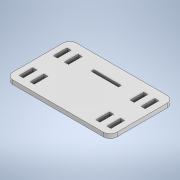
# Autodesk Inventor part: cambase
Saved by Autodesk Inventor 2020 (Build 240168000, 168)
## iProperties
Created: 2019-08-06
Part Number: cambase
Material: Generic
Document SubType Name: Modeling
Designer: n10208577
Density: 1 g/cm^3
Appearance: Default
Author: n10208577
Autodesk Inventor part; units mm, degrees
ref_plane "YZ Plane" through (0, 0, 0) normal (1, 0, 0) x (0, 1, 0)
ref_plane "XZ Plane" through (0, 0, 0) normal (0, 1, 0) x (-1, 0, 0)
ref_plane "XY Plane" through (0, 0, 0) normal (0, 0, 1) x (1, 0, 0)
sketch "Sketch1" plane through (0, 0, 0) normal (0, 1, 0) x (-1, 0, 0)
  line L0 (-21.1552, -13.1944) -> (-21.1552, -3.1944)
  line L1 (-21.1552, -3.1944) -> (-24.1552, -3.1944)
  line L2 (-24.1552, -3.1944) -> (-24.1552, -13.1944)
  line L3 (-24.1552, -13.1944) -> (-21.1552, -13.1944)
  line L4 (-21.1552, 11.8056) -> (-24.1552, 11.8056)
  line L5 (-24.1552, 11.8056) -> (-24.1552, 21.8056)
  line L6 (-24.1552, 21.8056) -> (-21.1552, 21.8056)
  line L7 (-21.1552, 21.8056) -> (-21.1552, 11.8056)
  line L8 (26.8448, -13.1944) -> (26.8448, -3.1944)
  line L9 (26.8448, -3.1944) -> (23.8448, -3.1944)
  line L10 (23.8448, -3.1944) -> (23.8448, -13.1944)
  line L11 (23.8448, -13.1944) -> (26.8448, -13.1944)
  line L12 (26.8448, 11.8056) -> (23.8448, 11.8056)
  line L13 (23.8448, 11.8056) -> (23.8448, 21.8056)
  line L14 (23.8448, 21.8056) -> (26.8448, 21.8056)
  line L15 (26.8448, 21.8056) -> (26.8448, 11.8056)
  line L16 (1.3448, -7.1944) -> (11.3448, -7.1944)
  line L17 (11.3448, -7.1944) -> (11.3448, -9.1944)
  line L18 (11.3448, -9.1944) -> (-8.6552, -9.1944)
  line L19 (-8.6552, -9.1944) -> (-8.6552, -7.1944)
  line L20 (-8.6552, -7.1944) -> (1.3448, -7.1944)
  line L21 (34.3448, -19.6944) -> (-31.6552, -19.6944)
  line L22 (-36.6552, -14.6944) -> (-36.6552, 21.8056)
  arc A0 (-36.6552, -14.6944) -> (-31.6552, -19.6944) centre (-31.6552, -14.6944) ccw
  arc A1 (-31.6552, 26.8056) -> (-36.6552, 21.8056) centre (-31.6552, 21.8056) ccw
  line L23 (-31.6552, 26.8056) -> (34.3448, 26.8056)
  arc A2 (39.3448, 21.8056) -> (34.3448, 26.8056) centre (34.3448, 21.8056) ccw
  line L24 (39.3448, 21.8056) -> (39.3448, -14.6944)
  arc A3 (34.3448, -19.6944) -> (39.3448, -14.6944) centre (34.3448, -14.6944) ccw
  line L25 (-29.1552, 11.8056) -> (-29.1552, 21.8056)
  line L26 (-29.1552, 21.8056) -> (-32.1552, 21.8056)
  line L27 (-32.1552, 21.8056) -> (-32.1552, 11.8056)
  line L28 (-32.1552, 11.8056) -> (-29.1552, 11.8056)
  line L29 (-29.1552, -13.1944) -> (-29.1552, -3.1944)
  line L30 (-29.1552, -3.1944) -> (-32.1552, -3.1944)
  line L31 (-32.1552, -3.1944) -> (-32.1552, -13.1944)
  line L32 (-32.1552, -13.1944) -> (-29.1552, -13.1944)
  line L33 (34.8448, -13.1944) -> (34.8448, -3.1944)
  line L34 (34.8448, -3.1944) -> (31.8448, -3.1944)
  line L35 (31.8448, -3.1944) -> (31.8448, -13.1944)
  line L36 (31.8448, -13.1944) -> (34.8448, -13.1944)
  line L37 (34.8448, 11.8056) -> (31.8448, 11.8056)
  line L38 (31.8448, 11.8056) -> (31.8448, 21.8056)
  line L39 (31.8448, 21.8056) -> (34.8448, 21.8056)
  line L40 (34.8448, 21.8056) -> (34.8448, 11.8056)
  constraints: 82 end point, 8 point on circle, 4 centre point
extrude "Extrusion1" add sketch "Sketch1" along normal blind 3
body "Solid1"
